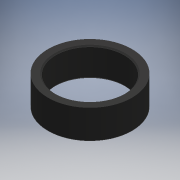
# Autodesk Inventor part: Distanziale lama
Saved by Autodesk Inventor 2018 (Build 220112000, 112)
## iProperties
Created: 2020-06-11
Part Number: Distanziale lama
Material: Generico
Document SubType Name: Modeling
Designer: Francesco
Density: 1 g/cm^3
Appearance: Gomma - Nero
Author: Francesco
Autodesk Inventor part; units mm, degrees
ref_plane "YZ Plane" through (0, 0, 0) normal (1, 0, 0) x (0, 1, 0)
ref_plane "XZ Plane" through (0, 0, 0) normal (0, 1, 0) x (-1, 0, 0)
ref_plane "XY Plane" through (0, 0, 0) normal (0, 0, 1) x (1, 0, 0)
sketch "Schizzo1" plane through (0, 0, 0) normal (0, 0, 1) x (1, 0, 0)
  circle A0 centre (0, 0) radius 14.25
  circle A1 centre (0, 0) radius 17.5
  dimension "d0" = 28.5
  dimension "d1" = 35
  constraints: 2 centre point, 2 coincident
  measures "d0" diameter of A0
  measures "d1" diameter of A1
extrude "Estrusione1" add sketch "Schizzo1" along normal blind 12
chamfer "Smusso1" distance 0.5 angle 45 2 edges at (-14.25, 0, 12) (-14.25, 0, 0)
